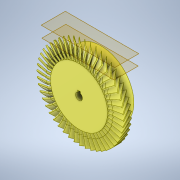
# Autodesk Inventor part: newRotor.48.2.6
Saved by Autodesk Inventor 2021.2 (Build 252289000, 289)
## iProperties
Created: 2021-05-16
Part Number: newRotor.48.2.6
Material: Generic
Document SubType Name: Modeling
Designer: Ryan
Density: 1 g/cm^3
Appearance: Smooth - Yellow
Author: Ryan
## iProperties of the stored document _3DPrint.ipt
Created: 2021-05-23
Part Number: _3DPrint
Material: Generic
Document SubType Name: Modeling
Designer: Ryan
Density: 1 g/cm^3
Appearance: Default
Author: Ryan
Autodesk Inventor part; units mm, degrees
ref_plane "YZ Plane" through (0, 0, 0) normal (1, 0, 0) x (0, 1, 0)
ref_plane "XY Plane" through (0, 0, 0) normal (0, 0, 1) x (1, 0, 0)
sketch "Sketch1" plane through (0, 0, 0) normal (0, 0, 1) x (1, 0, 0)
  circle A0 centre (0, 0) radius 33.02
  dimension "d0" = 66.04
  constraints: 1 centre point, 1 coincident
  measures "d0" diameter of A0
extrude "Extrusion1" add sketch "Sketch1" against normal blind 25.4 draft 11.31
ref_plane "Work Plane1" through (0, 38.1, 0) normal (0, 1, 0) x (-1, 0, 0)
sketch "Sketch2" plane through (0, 38.1, 0) normal (0, 1, 0) x (-1, 0, 0)
  line L0 (33.02, 0) -> (38.1, -25.4) projected
  line L1 (35.56, -12.7) -> (18.0568, -12.7)
  line L2 (33.02, 0) -> (-33.02, 0) projected
  line L3 (38.1, -25.4) -> (-38.1, -25.4) projected
  line L4 (0, -25.4) -> (0, 0)
  arc A0 (-4.774, -0.1017) -> (-5.6212, -1.563) centre (-5.1759, -0.8449) ccw
  arc A1 (2.7834, -11.1125) -> (-5.6212, -1.563) centre (-15.1085, -18.3861) ccw
  arc A2 (2.9588, -11.1125) -> (-4.774, -0.1017) centre (-12.9535, -14.0669) ccw
  line L5 (2.9588, -11.1125) -> (2.7834, -11.1125)
  point P0 (-3.0859, -11.9063)
  point P1 (3.0859, -11.9063)
  dimension "d4" = 0.7937
  constraints: 6 end point, 6 point on circle, 3 centre point, 2 horizontal, 2 midpoint, 1 symmetric about line, 1 vertical
  measures "d4" distance from line of point (-3.086, -11.906) L1
ref_plane "Work Plane2" through (0, 50.8, 0) normal (0, 1, 0) x (-1, 0, 0)
sketch "Sketch4" plane through (0, 50.8, 0) normal (0, 1, 0) x (-1, 0, 0)
  line L0 (38.1, -25.4) -> (-38.1, -25.4) projected
  line L1 (0, -25.4) -> (0, 0)
  arc A0 (-6.8775, -1.2594) -> (-7.5472, -2.251) centre (-7.1887, -1.7712) ccw
  line L2 (33.02, 0) -> (38.1, -25.4) projected
  line L3 (35.56, -12.7) -> (-35.56, -12.7)
  line L4 (-33.02, 0) -> (-38.1, -25.4) projected
  line L5 (6.5629, -11.1125) -> (0.9638, -11.1125)
  arc A1 (4.4574, -11.1125) -> (-7.5472, -2.251) centre (-30.972, -46.5467) ccw
  arc A2 (4.584, -11.1125) -> (-6.8775, -1.2594) centre (-30.9975, -40.9094) ccw
  line L6 (4.584, -11.1125) -> (4.4574, -11.1125)
  dimension "d47" = 1.5875
  constraints: 8 end point, 6 point on circle, 3 centre point, 3 midpoint, 2 point on line, 1 collinear, 1 horizontal, 1 vertical
  measures "d47" distance between parallel lines of L3 L5
sketch "Sketch5" plane through (0, 0, 0) normal (0, 0, 1) x (1, 0, 0)
  circle A0 centre (0, 0) radius 4
  line L0 (-1.5875, 5.5875) -> (1.5875, 5.5875)
  line L1 (1.5875, 5.5875) -> (1.5875, 2.4125)
  line L2 (1.5875, 2.4125) -> (-1.5875, 2.4125)
  line L3 (-1.5875, 2.4125) -> (-1.5875, 5.5875)
  line L4 (-1.5875, 5.5875) -> (1.5875, 2.4125) construction
  line L5 (1.5875, 5.5875) -> (-1.5875, 2.4125) construction
  point P0 (0, 4)
  point P1 (-1.5875, 3.6715)
  point P2 (1.5875, 3.6715)
  dimension "d38" = 8
  dimension "d39" = 3.175
  dimension "d40" = 3.175
  constraints: 12 end point, 2 midpoint, 2 parallel, 1 coincident, 1 horizontal, 1 perpendicular, 3 other
  measures "d39" distance of L1.end L2.end
  measures "d40" distance of L0.end L1.end
extrude "Extrusion3" cut sketch "Sketch5" against normal through all
sketch "Sketch6" plane through (0, 0, 0) normal (0, 0, 1) x (1, 0, 0)
  circle A0 centre (0, 0) radius 50.0063
  circle A1 centre (0, 0) radius 81.7071
  dimension "d43" = 100.0125
  constraints: 2 centre point, 2 coincident
  measures "d43" diameter of A0
extrude "Extrusion5" add sketch "Sketch2" against normal blind 7.62 contours A0 A2 L4 A1 | A2 L5 A1 L4
extrude "Extrusion6" add sketch "Sketch4" along normal blind 5.08 contours A1 A0 A2 L1 | L1 A2 L5 A1
loft "Loft4" add section 1 edges at (-0.2909, 38.1, -4.7654) (5.9068, 38.1, -0.4211) (0.6101, 38.1, -5.6259) (-2.8711, 38.1, -11.1125) section 2 edges at (1.2132, 50.8, -6.2324) (7.6851, 50.8, -1.4359) (0.7429, 50.8, -5.7163) (-4.5207, 50.8, -11.1125)
pattern_circular "Circular Pattern7" count 48 over 360 about axis through (0, 0, -10) along (0, 0, 1) of "Extrusion5", "Loft4", "Extrusion6"
extrude "Extrusion7" cut sketch "Sketch6" against normal through all
body "Solid1"
